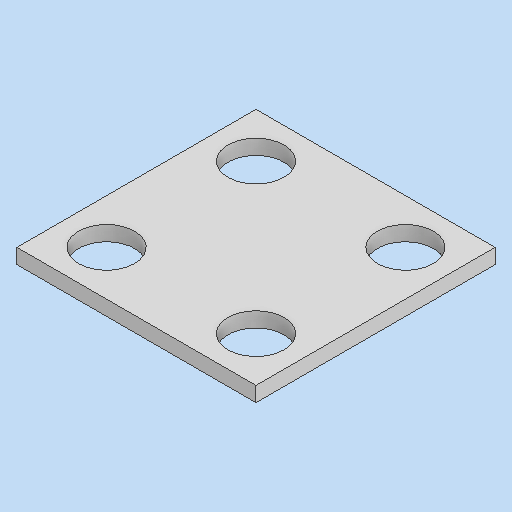
# Autodesk Inventor part: 零件1
Saved by Autodesk Inventor 2026.2 (Build 302298010, 298A)
## iProperties
Created: 2026-03-16
Part Number: 零件1
Material: 常规
Document SubType Name: Modeling
Designer: liu
Density: 1 g/cm^3
Appearance: 默认
Author: liu
Autodesk Inventor part; units mm, degrees
ref_plane "YZ Plane" through (0, 0, 0) normal (1, 0, 0) x (0, 1, 0)
ref_plane "XZ Plane" through (0, 0, 0) normal (0, 1, 0) x (-1, 0, 0)
ref_plane "XY Plane" through (0, 0, 0) normal (0, 0, 1) x (1, 0, 0)
sketch "草图1" plane through (0, 0, 0) normal (0, 1, 0) x (-1, 0, 0)
  line L0 (80, 80) -> (0, 80)
  line L1 (0, 80) -> (0, 0)
  line L2 (0, 0) -> (80, 0)
  line L3 (80, 0) -> (80, 80)
  dimension "d1" = 80
  dimension "d2" = 80
  constraints: 8 end point, 2 parallel, 1 coincident, 1 horizontal, 1 perpendicular
  measures "d1" distance of L1.end L2.end
  measures "d2" distance of L2.end L0.start
extrude "拉伸1" add sketch "草图1" along normal blind 5
sketch "草图2" plane through (0, 5, 0) normal (0, 1, 0) x (1, 0, 0)
  circle A0 centre (-65, -65) radius 9.3759
  line L0 (-80, 0) -> (-80, -80) projected
  line L1 (-80, -80) -> (0, -80) projected
  circle A1 centre (-65, -15) radius 9.3759
  circle A2 centre (-15, -15) radius 9.3759
  circle A3 centre (-15, -65) radius 9.3759
  point P0 (0, 0)
  dimension "d5" = 15
  dimension "d6" = 15
  dimension "d9" = 50
  dimension "d16" = 50
  dimension "d23" = 50
  constraints: 4 centre point, 2 vertical, 1 horizontal, 6 other
  measures "d5" distance from line of L0 A0.centre
  measures "d6" distance from line of L1 A0.centre
  measures "d9" distance of A0.centre A1.centre
  measures "d16" distance of A1.centre A2.centre
  measures "d23" distance of A2.centre A3.centre
extrude "拉伸2" cut sketch "草图2" against normal blind 5
